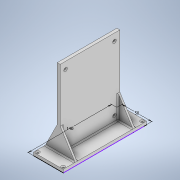
# Autodesk Inventor part: support
Saved by Autodesk Inventor 2021 (Build 250183000, 183)
## iProperties
Created: 2021-03-14
Part Number: support
Material: Generic
Document SubType Name: Modeling
Designer: awitc
Density: 1 g/cm^3
Appearance: Default
Author: awitc
Autodesk Inventor part; units mm, degrees
ref_plane "YZ Plane" through (0, 0, 0) normal (1, 0, 0) x (0, 1, 0)
ref_plane "XZ Plane" through (0, 0, 0) normal (0, 1, 0) x (-1, 0, 0)
ref_plane "XY Plane" through (0, 0, 0) normal (0, 0, 1) x (1, 0, 0)
sketch "Sketch1" plane through (0, 0, 0) normal (0, 1, 0) x (-1, 0, 0)
  line L0 (0, 0) -> (46, 0)
  line L1 (0, -135) -> (0, 0)
  line L2 (0, 0) -> (50, 0)
  line L3 (50, 0) -> (50, -140)
  line L4 (50, -140) -> (0, -140)
  line L5 (0, -140) -> (0, 0)
  dimension "d36" = 50
  dimension "d37" = 140
  constraints: 12 end point, 2 horizontal, 2 parallel, 1 perpendicular
  measures "d36" distance of L3.end L4.end
  measures "d37" distance of L2.end L3.end
extrude "Extrusion1" add sketch "Sketch1" along normal blind 5
sketch "Sketch2" plane through (0, 5, 0) normal (0, 1, 0) x (1, 0, 0)
  line L0 (0, 2.5) -> (17, 2.5) construction
  circle A0 centre (-3.75, 136.25) radius 1.5
  circle A1 centre (-46.25, 136.25) radius 1.5
  line L1 (0, 0) -> (-3.75, 0)
  circle A2 centre (-3.75, 3.75) radius 1.5
  circle A3 centre (-46.25, 3.75) radius 1.5
  point P0 (0, 135)
  point P1 (-50, 140)
  point P2 (0, 140)
  dimension "d103" = 3
  dimension "d106" = 3
  dimension "d109" = 3
  dimension "d110" = 3
  constraints: 4 centre point, 4 end point, 2 horizontal
  measures "d103" diameter of A0
  measures "d106" diameter of A1
  measures "d109" diameter of A2
  measures "d110" diameter of A3
extrude "Extrusion4" cut sketch "Sketch2" against normal through all
sketch "Sketch3" plane through (0, 5, 0) normal (0, 1, 0) x (1, 0, 0)
  line L0 (0, 0) -> (0, 140) projected
  line L1 (0, 70) -> (-25, 70)
  line L2 (0, 140) -> (-50, 140) projected
  line L3 (-25, 70) -> (-30, 70)
  line L4 (-30, 115) -> (-30, 70)
  line L5 (-30, 25) -> (-30, 70)
  line L6 (-30, 115) -> (-25, 115)
  line L7 (-25, 115) -> (-25, 25)
  line L8 (-25, 25) -> (-30, 25)
  line L9 (-30, 25) -> (-30, 115)
  line L10 (-25, 115) -> (-30, 115)
  line L11 (-30, 115) -> (-30, 120)
  line L12 (-30, 120) -> (-25, 120)
  line L13 (-25, 120) -> (-25, 115)
  line L14 (-25, 25) -> (-30, 25)
  line L15 (-30, 25) -> (-30, 20)
  line L16 (-30, 20) -> (-25, 20)
  line L17 (-25, 20) -> (-25, 25)
  dimension "d55" = 5
  dimension "d56" = 5
  constraints: 32 end point, 7 parallel, 4 horizontal, 3 perpendicular, 1 midpoint, 1 point on line
  measures "d55" distance of L10.end L11.end
  measures "d56" distance of L15.end L14.end
extrude "Extrusion5" add sketch "Sketch3" along normal blind 130
sketch "Sketch5" plane through (-30, 5, -120) normal (-1, 0, 0) x (0, 0, 1)
  line L0 (100, 0) -> (100, 130) projected
  line L1 (120, 0) -> (-20, 0) projected
  circle A0 centre (9.0002, 118) radius 1.5
  circle A1 centre (91.0002, 118) radius 1.5
  circle A2 centre (91.0002, 10) radius 1.5
  circle A3 centre (9.0002, 10) radius 1.5
  point P0 (120, -5)
  dimension "d62" = 3
  dimension "d63" = 3
  dimension "d64" = 3
  dimension "d65" = 3
  constraints: 4 centre point
  measures "d62" diameter of A0
  measures "d63" diameter of A1
  measures "d64" diameter of A2
  measures "d65" diameter of A3
extrude "Extrusion6" cut sketch "Sketch5" against normal up to surface (5 mm away)
sketch "Sketch6" plane through (-30, 5, -120) normal (-1, 0, 0) x (0, 0, 1)
  line L0 (0, 0) -> (3, 0)
  line L1 (3, 0) -> (3, 40)
  line L2 (3, 40) -> (0, 40)
  line L3 (0, 40) -> (0, 0)
  line L4 (100, 0) -> (0, 0) projected
  line L5 (100, 0) -> (97, 0)
  line L6 (97, 0) -> (97, 40)
  line L7 (97, 40) -> (100, 40)
  line L8 (100, 40) -> (100, 0)
  point P0 (120, -5)
  dimension "d68" = 3
  dimension "d69" = 40
  dimension "d70" = 3
  dimension "d71" = 40
  constraints: 16 end point, 4 parallel, 2 horizontal, 2 perpendicular
  measures "d68" distance of L2.end L1.end
  measures "d69" distance of L1.end L0.end
  measures "d70" distance of L6.end L7.end
  measures "d71" distance of L5.end L6.end
extrude "Extrusion7" add sketch "Sketch6" along normal blind 20 and the other way blind 30
sketch "Sketch7" plane through (0, 5, -120) normal (0, 0, -1) x (-1, 0, 0)
  line L0 (0, 40) -> (25, 40) projected
  line L1 (50, 0) -> (50, 40) projected
  line L2 (0, 40) -> (50, 40)
  line L3 (50, 40) -> (50, 0)
  line L4 (50, 0) -> (0, 0)
  line L5 (0, 0) -> (0, 40)
  line L6 (50, 0) -> (0, 0) projected
  line L7 (25, 40) -> (0, 0)
  line L8 (30, 40) -> (50, 0)
  point P0 (0, -5)
  constraints: 12 end point, 2 parallel, 1 horizontal, 1 perpendicular
sketch "Sketch8" plane through (-50, 5, -20) normal (0, 0, 1) x (1, 0, 0)
  line L0 (20, 40) -> (0, 40) projected
  line L1 (50, 40) -> (50, 0) projected
  line L2 (0, 40) -> (50, 40)
  line L3 (50, 40) -> (50, 0)
  line L4 (50, 0) -> (0, 0)
  line L5 (0, 0) -> (0, 40)
  line L6 (20, 40) -> (0, 0)
  line L7 (50, 40) -> (25, 40) projected
  line L8 (25, 40) -> (50, 0)
  point P0 (50, -5)
  constraints: 12 end point, 2 parallel, 1 horizontal, 1 perpendicular
extrude "Extrusion8" cut sketch "Sketch8" against normal up to surface (3 mm away) contours L6 L5 L0 | L2 L1 L8
extrude "Extrusion9" cut sketch "Sketch7" against normal up to surface (3 mm away) contours L0 L7 L5 | L2 L1 L8
fillet "Fillet1" radius 2 8 edges at (-30, 5, -70) (-25, 5, -70) (-12.5, 5, -117) (-40, 5, -117) (-40, 5, -23) (-12.5, 5, -23) (-25, 5, -20) (-25, 5, -120)
thread "Thread5" size "M3x0.5" class "6H" standard "ANSI Metric M Profile" full length
thread "Thread6" size "M3x0.5" class "6H" standard "ANSI Metric M Profile" full length
thread "Thread7" size "M3x0.5" class "6H" standard "ANSI Metric M Profile" full length
thread "Thread8" size "M3x0.5" class "6H" standard "ANSI Metric M Profile" full length
fillet "Fillet2" radius 2 8 edges at (-30.5858, 5.5858, -23.5858) (-30, 26, -23) (-30.5858, 5.5858, -116.4142) (-30, 26, -117) (-24.4142, 5.5858, -116.4142) (-25, 26, -117) (-24.4142, 5.5858, -23.5858) (-25, 26, -23)
chamfer "Chamfer1" distance 1.5 angle 45 8 edges at (-25, 123, -30.4998) (-25, 123, -112.4998) (-25, 15, -112.4998) (-25, 15, -30.4998) (-5.25, 5, -136.25) (-47.75, 5, -136.25) (-5.25, 5, -3.75) (-47.75, 5, -3.75)
chamfer_without_effect "Chamfer2"
thread "Thread13" size "M3x0.5" class "6H" standard "ANSI Metric M Profile" full length
thread "Thread14" size "M3x0.5" class "6H" standard "ANSI Metric M Profile" full length
thread "Thread15" size "M3x0.5" class "6H" standard "ANSI Metric M Profile" full length
thread "Thread16" size "M3x0.5" class "6H" standard "ANSI Metric M Profile" full length
body "Solid1"
